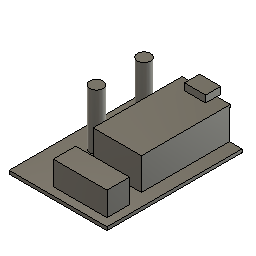
F000120 - Protoype Ingun Switch Case Assembly v8 (Autodesk Fusion 360 archive; units mm, degrees)
design "F000117 - Prototype Ingun Switch Breakout"
Autodesk Fusion 360 part; units mm, degrees
sketch "Sketch1" plane through (0, 0, 0) normal (0, 1, 0) x (1, 0, 0)
  line L0 (0, 0) -> (37, 0)
  line L1 (37, 0) -> (37, 51)
  line L2 (37, 51) -> (0, 51)
  line L3 (0, 51) -> (0, 0)
  line L4 (13.7, 3) -> (34, 3)
  line L5 (34, 3) -> (34, 11.5)
  line L6 (34, 11.5) -> (13.7, 11.5)
  line L7 (13.7, 11.5) -> (13.7, 3)
  line L8 (14, 17.75) -> (32.25, 17.75)
  line L9 (32.25, 17.75) -> (32.25, 51.35)
  line L10 (32.25, 51.35) -> (14, 51.35)
  line L11 (14, 51.35) -> (14, 17.75)
  line L12 (19.125, 47.15) -> (27.125, 47.15)
  line L13 (27.125, 47.15) -> (27.125, 52.85)
  line L14 (27.125, 52.85) -> (19.125, 52.85)
  line L15 (19.125, 52.85) -> (19.125, 47.15)
  circle A0 centre (9.5, 41.5) radius 2.5
  circle A1 centre (9.5, 23.5) radius 2.5
  dimension "d1" = 37
  dimension "d2" = 51
  dimension "d3" = 3
  dimension "d4" = 3
  dimension "d5" = 20.3
  dimension "d6" = 8.5
  dimension "d7" = 6.25
  dimension "d8" = 18.25
  dimension "d9" = 4.75
  dimension "d10" = 33.6
  dimension "d11" = 5.7
  dimension "d12" = 8
  dimension "d13" = 5.125
  dimension "d15" = 1.5
  dimension "d16" = 9.5
  dimension "d17" = 9.5
  dimension "d18" = 5
  dimension "d19" = 27.5
  constraint horizontal L0
  constraint vertical L1
  constraint horizontal L2
  constraint vertical L3
  constraint coincident L0.start L3.end
  constraint horizontal L4
  constraint vertical L5
  constraint horizontal L6
  constraint vertical L7
  constraint horizontal L8
  constraint vertical L9
  constraint horizontal L10
  constraint vertical L11
  constraint horizontal L12
  constraint vertical L13
  constraint horizontal L14
  constraint vertical L15
  constraint equal A0 A1
  constraint vertical A0.centre A1.centre
  measures "d1" distance of L0.start L0.end
  measures "d2" distance of L0.start L2.end
  measures "d3" distance of L0 L4
  measures "d4" distance of L1 L5
  measures "d5" distance of L4.start L4.end
  measures "d6" distance of L4.start L6.end
  measures "d7" distance of L6 L8
  measures "d8" distance of L8.start L8.end
  measures "d9" distance of L1 L9
  measures "d10" distance of L8.end L9.end
  measures "d11" distance of L12.start L14.end
  measures "d12" distance of L13.end L14.end
  measures "d13" distance of L11 L15
  measures "d15" distance of L10 L14
  measures "d16" distance of L2 A0.centre
  measures "d17" distance of L3 A0.centre
  measures "d18" diameter of A0
  measures "d19" distance of L2 A1.centre
extrude "Extrude1" add sketch "Sketch1" against normal blind 1.25 contours L0 L1 L2 L3 L8 L9 L11 | L2 L8 L9 L11 L12 L13 L15 | L2 L12 L13 L15 | L4 L5 L6 L7 | A0 | A1
extrude "Extrude2" add sketch "Sketch1" along normal blind 9 contours L4 L5 L6 L7
extrude "Extrude3" add sketch "Sketch1" along normal blind 11 contours L2 L8 L9 L11 L12 L13 L15 | L2 L12 L13 L15
sketch "Sketch3" plane through (0, 11, 0) normal (0, 1, 0) x (-1, 0, 0)
  line L0 (-32.25, -51) -> (-14, -51)
  line L1 (-14, -51) -> (-14, -17.75)
  line L2 (-14, -17.75) -> (-32.25, -17.75)
  line L3 (-32.25, -17.75) -> (-32.25, -51)
  line L4 (-14, -17.75) -> (-32.25, -17.75)
  line L5 (-32.25, -17.75) -> (-32.25, -51.35)
  line L6 (-32.25, -51.35) -> (-14, -51.35)
  line L7 (-14, -51.35) -> (-14, -17.75)
  dimension "d26" = 33.6
  dimension "d27" = 18.25
  constraint horizontal L4
  constraint vertical L5
  constraint horizontal L6
  constraint vertical L7
  constraint coincident L1.end L2.start
  measures "d26" distance of L2.end L5.end
  measures "d27" distance of L5.end L6.end
extrude "Extrude4" add sketch "Sketch3" along normal blind 1
sketch "Sketch4" plane through (0, 12, 0) normal (0, 1, 0) x (-1, 0, 0)
  line L0 (-14, -51.35) -> (-14, -17.75)
  line L1 (-14, -17.75) -> (-32.25, -17.75)
  line L2 (-32.25, -17.75) -> (-32.25, -51.35)
  line L3 (-32.25, -51.35) -> (-14, -51.35)
  line L4 (-19.125, -47.15) -> (-27.125, -47.15)
  line L5 (-27.125, -47.15) -> (-27.125, -52.85)
  line L6 (-27.125, -52.85) -> (-19.125, -52.85)
  line L7 (-19.125, -52.85) -> (-19.125, -47.15)
  line L8 (-32.25, -51.35) -> (-14, -51.35)
  dimension "d30" = 5.125
  dimension "d31" = 8
  dimension "d32" = 5.7
  dimension "d33" = 1.5
  constraint horizontal L4
  constraint vertical L5
  constraint horizontal L6
  constraint vertical L7
  measures "d30" distance of L0.start L7
  measures "d31" distance of L5.end L6.end
  measures "d32" distance of L4.start L6.end
  measures "d33" distance of L6 L8
extrude "Extrude5" add sketch "Sketch4" along normal blind 2.6 contours L3 L5 L6 L7 L8 | L3 L4 L5 L7 L8
extrude "Extrude6" add sketch "Sketch1" along normal blind 21 contours A0 | A1
sketch "Sketch6" plane through (0, -1.25, 0) normal (0, -1, 0) x (1, 0, 0)
  line L0 (0, 0) -> (0, -51)
  line L1 (0, -51) -> (37, -51)
  line L2 (37, -51) -> (37, 0)
  line L3 (37, 0) -> (0, 0)
  line L4 (4, -4) -> (33, -4)
  line L5 (33, -4) -> (33, -49)
  line L6 (33, -49) -> (4, -49)
  line L7 (4, -49) -> (4, -4)
  dimension "d38" = 2
  dimension "d39" = 4
  dimension "d41" = 4
  dimension "d42" = 4
  dimension "d45" = 29
  dimension "d46" = 45
  constraint horizontal L4
  constraint vertical L5
  constraint horizontal L6
  constraint vertical L7
  measures "d38" distance of L1 L6
  measures "d39" distance of L0 L7
  measures "d41" distance of L2 L5
  measures "d42" distance of L3 L4
  measures "d45" distance of L4.start L4.end
  measures "d46" distance of L4.start L6.end
extrude "Extrude7" [suppressed]

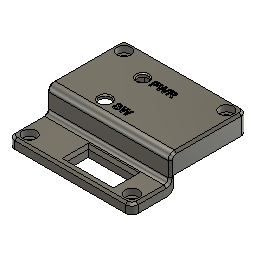
design "F000119 - Case Top"
Autodesk Fusion 360 part; units mm, degrees
sketch "Sketch1" plane through (0, 0, 0) normal (0, 1, 0) x (1, 0, 0)
  line L0 (0, 0) -> (59, 0)
  line L1 (59, 0) -> (59, 56.2)
  line L2 (59, 56.2) -> (0, 56.2)
  line L3 (0, 56.2) -> (0, 0)
  line L4 (23.85, 14.25) -> (45.85, 14.25)
  line L5 (45.85, 14.25) -> (45.85, 4.25)
  line L6 (45.85, 4.25) -> (23.85, 4.25)
  line L7 (23.85, 4.25) -> (23.85, 14.25)
  line L8 (0, 18.25) -> (59, 18.25)
  line L9 (0, 19.85) -> (59, 19.85)
  dimension "d1" = 59
  dimension "d2" = 56.2
  dimension "d3" = 13.15
  dimension "d4" = 10
  dimension "d5" = 22
  dimension "d6" = 4.25
  dimension "d11" = 4
  dimension "d12" = 1.6
  constraint horizontal L0
  constraint vertical L1
  constraint horizontal L2
  constraint vertical L3
  constraint coincident L0.start L3.end
  constraint horizontal L4
  constraint vertical L5
  constraint horizontal L6
  constraint vertical L7
  constraint coincident L3 L8.start
  constraint coincident L1 L8.end
  constraint perpendicular L1 L8
  constraint coincident L3 L9.start
  constraint coincident L1 L9.end
  constraint perpendicular L1 L9
  measures "d1" distance of L0.start L0.end
  measures "d2" distance of L0.start L2.end
  measures "d3" distance of L1 L5
  measures "d4" distance of L4.end L5.end
  measures "d5" distance of L4.start L4.end
  measures "d11" distance of L4 L8
  measures "d12" distance of L8 L9
  measures "d24" distance of L0.start
  measures "d34" distance of L0.start
  measures "d51" distance of L0.start
extrude "Extrude1" add sketch "Sketch1" against normal blind 4.6 contours L0 L1 L3 L8 | L1 L3 L8 L9
extrude "Extrude2" add sketch "Sketch1" along normal blind 10.45 contours L1 L3 L8 L9
sketch "Sketch2" plane through (0, 10.45, 0) normal (0, 1, 0) x (-1, 0, 0)
  line L0 (0, -18.25) -> (-59, -18.25)
  line L1 (-59, -18.25) -> (-59, -19.85)
  line L2 (-59, -19.85) -> (0, -19.85)
  line L3 (0, -19.85) -> (0, -18.25)
  line L4 (0, -18.25) -> (-59, -18.25)
  line L5 (-59, -18.25) -> (-59, -55.2)
  line L6 (-59, -55.2) -> (0, -55.2)
  line L7 (0, -55.2) -> (0, -18.25)
  dimension "d15" = 36.95
  dimension "d16" = 59
  constraint horizontal L4
  constraint vertical L5
  constraint horizontal L6
  constraint vertical L7
  constraint coincident L0.start L3.end
  measures "d15" distance of L0.start L6.end
  measures "d16" distance of L5.end L6.end
extrude "Extrude3" add sketch "Sketch2" along normal blind 1.6
fillet "Fillet1" radius 2 1 edges at (29.5, 0, -18.25)
fillet "Fillet2" radius 3 1 edges at (29.5, -4.6, -19.85)
fillet "Fillet3" radius 3 1 edges at (29.5, 12.05, -18.25)
sketch "Sketch3" plane through (0, 10.45, 0) normal (0, -1, 0) x (1, 0, 0)
  line L0 (59, -19.85) -> (0, -19.85)
  line L1 (0, -19.85) -> (0, -55.2)
  line L2 (0, -55.2) -> (59, -55.2)
  line L3 (59, -55.2) -> (59, -19.85)
  line L4 (57.4, -53.6) -> (1.6, -53.6)
  line L5 (1.6, -53.6) -> (1.6, -19.85)
  line L6 (1.6, -19.85) -> (57.4, -19.85)
  line L7 (57.4, -19.85) -> (57.4, -53.6)
  line L8 (1.6, -53.6) -> (1.6, -55.2)
  line L9 (57.4, -53.6) -> (57.4, -55.2)
  line L10 (3.2, -53.6) -> (3.2, -19.85)
  line L11 (55.8, -19.85) -> (55.8, -53.6)
  line L12 (3.2, -52) -> (55.8, -52)
  line L13 (44.25, -52) -> (44.25, -53.6)
  line L14 (24, -52) -> (24, -53.6)
  dimension "d23" = 1.6
  dimension "d24" = 1.6
  dimension "d25" = 1.6
  dimension "d73" = 1.6
  dimension "d74" = 1.6
  dimension "d77" = 1.6
  dimension "d83" = 22.4
  dimension "d84" = 13.15
  constraint horizontal L4
  constraint vertical L5
  constraint horizontal L6
  constraint vertical L7
  constraint horizontal L0.start L6.end
  constraint coincident L2 L8.end
  constraint perpendicular L2 L8
  constraint coincident L2 L9.end
  constraint perpendicular L2 L9
  constraint parallel L5 L10
  constraint parallel L7 L11
  constraint coincident L0 L10.end
  constraint coincident L4 L10.start
  constraint coincident L6 L11.start
  constraint coincident L4 L11.end
  constraint coincident L10 L12.start
  constraint coincident L11 L12.end
  constraint perpendicular L11 L12
  constraint coincident L12 L13.start
  constraint coincident L4 L13.end
  constraint perpendicular L4 L13
  constraint coincident L12 L14.start
  constraint coincident L4 L14.end
  constraint perpendicular L4 L14
  measures "d23" distance of L3 L7
  measures "d24" distance of L1 L5
  measures "d25" distance of L2 L4
  measures "d73" distance of L5 L10
  measures "d74" distance of L7 L11
  measures "d77" distance of L4 L12
  measures "d83" distance of L4.end L14
  measures "d84" distance of L4.start L13
extrude "Extrude4" add sketch "Sketch3" along normal blind 7.7 contours L0 L2 L3 L7 L9 | L0 L1 L2 L5 L8
extrude "Extrude10" add sketch "Sketch3" along normal blind 8.7 contours L0 L4 L6 L7 L11 | L0 L4 L5 L6 L10 | L4 L11 L12 L13 | L4 L10 L12 L14
sketch "Sketch4" plane through (0, 0, -55.2) normal (0, 0, -1) x (-1, 0, 0)
  line L0 (-57.4, 10.45) -> (-1.6, 10.45)
  line L1 (-1.6, 10.45) -> (-1.6, 2.75)
  line L2 (-1.6, 2.75) -> (0, 2.75)
  line L3 (0, 2.75) -> (0, 12.05)
  line L4 (0, 12.05) -> (-59, 12.05)
  line L5 (-59, 12.05) -> (-59, 2.75)
  line L6 (-59, 2.75) -> (-57.4, 2.75)
  line L7 (-57.4, 2.75) -> (-57.4, 10.45)
  line L8 (-59, 12.05) -> (0, 12.05)
  line L9 (0, 12.05) -> (0, 2.75)
  line L10 (0, 2.75) -> (-59, 2.75)
  line L11 (-59, 2.75) -> (-59, 12.05)
  line L12 (-38.25, 12.05) -> (-30, 12.05)
  line L13 (-30, 12.05) -> (-30, 2.75)
  line L14 (-30, 2.75) -> (-38.25, 2.75)
  line L15 (-38.25, 2.75) -> (-38.25, 12.05)
  line L16 (-38.25, 5.95) -> (-30, 5.95)
  dimension "d28" = 20.75
  dimension "d29" = 30
  dimension "d40" = 3.2
  constraint horizontal L8
  constraint vertical L9
  constraint horizontal L10
  constraint vertical L11
  constraint coincident L2.end L3.start
  constraint coincident L4.end L5.start
  constraint horizontal L12
  constraint vertical L13
  constraint horizontal L14
  constraint vertical L15
  constraint coincident L10 L13.end
  constraint coincident L8 L12.start
  constraint coincident L15 L16.start
  constraint coincident L13 L16.end
  constraint perpendicular L13 L16
  measures "d28" distance of L11 L15
  measures "d29" distance of L9 L13
  measures "d40" distance of L14 L16
extrude "Extrude5" add sketch "Sketch4" against normal blind 1.6 contours L0 L7 L10 L15 | L0 L1 L10 L13
sketch "Sketch5" plane through (0, 12.05, 0) normal (0, 1, 0) x (-1, 0, 0)
  line L0 (0, -21.25) -> (-59, -21.25)
  line L1 (-59, -21.25) -> (-59, -55.2)
  line L2 (-59, -55.2) -> (0, -55.2)
  line L3 (0, -55.2) -> (0, -21.25)
  circle A0 centre (-20.5, -25.6) radius 2.75
  circle A1 centre (-20.5, -43.6) radius 2.6
  dimension "d32" = 5.5
  dimension "d33" = 5.2
  dimension "d34" = 20.5
  dimension "d36" = 29.6
  dimension "d39" = 18
  constraint vertical A0.centre A1.centre
  measures "d32" diameter of A0
  measures "d33" diameter of A1
  measures "d34" distance of L3 A1.centre
  measures "d36" distance of L2 A0.centre
  measures "d39" distance of A0.centre A1.centre
extrude "Extrude6" cut sketch "Sketch5" against normal blind 19 contours A0 | A1
extrude "Extrude7" add sketch "Sketch4" against normal blind 1.6 contours L0 L13 L15 L16
sketch "Sketch6" plane through (0, 10.45, 0) normal (0, -1, 0) x (1, 0, 0)
  line L0 (24, -53.6) -> (44.25, -53.6)
  line L1 (55.8, -19.85) -> (3.2, -19.85)
  circle A0 centre (20.5, -43.6) radius 2.6
  circle A1 centre (20.5, -25.6) radius 2.75
  line L2 (1.6, -45.2) -> (10, -45.2)
  line L3 (10, -45.2) -> (10, -53.6)
  line L4 (57.4, -45.2) -> (49, -45.2)
  line L5 (49, -45.2) -> (49, -53.6)
  line L6 (44.25, -53.6) -> (44.25, -52)
  line L7 (44.25, -52) -> (55.8, -52)
  line L8 (55.8, -52) -> (55.8, -19.85)
  line L9 (3.2, -19.85) -> (3.2, -52)
  line L10 (3.2, -52) -> (24, -52)
  line L11 (24, -52) -> (24, -53.6)
  dimension "d43" = 8.4
  dimension "d44" = 8.4
  dimension "d45" = 8.4
  dimension "d46" = 8.4
  constraint coincident L0 L3.end
  constraint perpendicular L0 L3
  constraint coincident L0 L5.end
  constraint perpendicular L0 L5
  measures "d43" distance of L2.end L3.end
  measures "d44" distance of L2.start L2.end
  measures "d45" distance of L4.start L4.end
  measures "d46" distance of L4.end L5.end
extrude "Extrude8" add sketch "Sketch6" along normal blind 8.7 contours L2 L3 L9 L10 | L4 L5 L7 L8
fillet "Fillet4" radius 3 8 edges at (10, 6.1, -52) (10, 6.1, -45.2) (3.2, 6.1, -45.2) (49, 6.1, -52) (49, 6.1, -45.2) (55.8, 6.1, -45.2) (55.8, 6.1, -19.85) (3.2, 6.1, -19.85)
sketch "Sketch7" plane through (0, 12.05, 0) normal (0, 1, 0) x (-1, 0, 0)
  circle A0 centre (-20.5, -25.6) radius 2.75
  circle A1 centre (-20.5, -43.6) radius 2.6
  line L0 (0, -21.25) -> (-59, -21.25)
  line L1 (-59, -21.25) -> (-59, -55.2)
  line L2 (-59, -55.2) -> (0, -55.2)
  line L3 (0, -55.2) -> (0, -21.25)
  point P0 (-5, -50.2)
  point P1 (-54, -50.2)
  dimension "d50" = 5
  dimension "d51" = 5
  dimension "d52" = 5
  constraint horizontal P0 P1
  measures "d50" distance of L2 P0
  measures "d51" distance of L3 P0
  measures "d52" distance of L1 P1
sketch "Sketch8" plane through (0, 0, 0) normal (0, 1, 0) x (-1, 0, 0)
  line L0 (-59, -16.25) -> (0, -16.25)
  line L1 (0, -16.25) -> (0, 0)
  line L2 (0, 0) -> (-59, 0)
  line L3 (-59, 0) -> (-59, -16.25)
  line L4 (-45.85, -4.25) -> (-23.85, -4.25)
  line L5 (-23.85, -4.25) -> (-23.85, -14.25)
  line L6 (-23.85, -14.25) -> (-45.85, -14.25)
  line L7 (-45.85, -14.25) -> (-45.85, -4.25)
  point P0 (-5, -5)
  point P1 (-54, -5)
  dimension "d58" = 5
  dimension "d59" = 5
  dimension "d60" = 5
  constraint horizontal P0 P1
  measures "d58" distance of L1 P0
  measures "d59" distance of L2 P0
  measures "d60" distance of L3 P1
hole "Hole1" at (5, 12.05, -50.2) at (54, 12.05, -50.2) direction (0, -1, 0) diameter 3.4 depth 14 tip angle 180 counterbore diameter 6.5 counterbore depth 3
hole "Hole2" at (5, 0, -5) at (54, 0, -5) direction (0, -1, 0) diameter 3.4 depth 10 tip angle 180 counterbore diameter 6.5 counterbore depth 3
fillet "Fillet5" radius 3 4 edges at (59, 7.4, -55.2) (0, 7.4, -55.2) (0, -2.3, 0) (59, -2.3, 0)
chamfer "Chamfer1" distance 1 angle 45 16 edges at (0, 11.1713, -19.1287) (0, 5.525, -18.25) (0, 0.5858, -17.6642) (0, 0, -9.625) (0.8787, 0, -0.8787) (29.5, 0, 0) (58.1213, 0, -0.8787) (59, 0, -9.625) (59, 0.5858, -17.6642) (59, 5.525, -18.25) (59, 11.1713, -19.1287) (59, 12.05, -36.725) (58.1213, 12.05, -54.3213) (29.5, 12.05, -55.2) (0.8787, 12.05, -54.3213) (0, 12.05, -36.725)
chamfer "Chamfer2" distance 1.25 angle 45 4 edges at (34.85, 0, -4.25) (23.85, 0, -9.25) (34.85, 0, -14.25) (45.85, 0, -9.25)
fillet "Fillet6" radius 0.5 2 edges at (22.9241, 12.05, -42.6598) (23.0639, 12.05, -24.6056)
sketch "Sketch9" plane through (0, 12.05, 0) normal (0, 1, 0) x (-1, 0, 0)
  circle A0 centre (-20.5, -43.6) radius 3.1
  circle A1 centre (-5, -50.2) radius 3.25
  circle A2 centre (-54, -50.2) radius 3.25
  line L0 (-58, -21.25) -> (-58, -52.2)
  arc A3 (-58, -52.2) -> (-56, -54.2) centre (-56, -52.2) ccw
  line L1 (-56, -54.2) -> (-3, -54.2)
  arc A4 (-3, -54.2) -> (-1, -52.2) centre (-3, -52.2) ccw
  line L2 (-1, -52.2) -> (-1, -21.25)
  line L3 (-1, -21.25) -> (-58, -21.25)
  circle A5 centre (-20.5, -25.6) radius 3.25
  line L4 (-25, -42) -> (-36.1861, -41.9973) construction
  line L5 (-36.1861, -41.9973) -> (-36.1872, -46.8542) construction
  line L6 (-36.1872, -46.8542) -> (-25.0012, -46.8569) construction
  line L7 (-25.0012, -46.8569) -> (-25, -42) construction
  line L8 (-25, -23.9666) -> (-32.7185, -23.9597) construction
  line L9 (-32.7185, -23.9597) -> (-32.7229, -28.7859) construction
  line L10 (-32.7229, -28.7859) -> (-25.0043, -28.7928) construction
  line L11 (-25.0043, -28.7928) -> (-25, -23.9666) construction
  text T0 "PWR" font "Arial" height 4.8569 bold align ink ink in box 0 x 0 at (-25, -42) x (-1, 0.000243) y (-0.000243, -1) spacing 1 height is em
  text T1 "SW" font "Arial" height 4.8262 bold align ink ink in box 0 x 0 at (-25, -23.9666) x (-1, 0.000895) y (-0.000895, -1) spacing 1 height is em
  constraint perpendicular L4 L5
  constraint parallel L4 L6
  constraint parallel L5 L7
  constraint perpendicular L8 L9
  constraint parallel L8 L10
  constraint parallel L9 L11
  constraint vertical L4.start L8.start
extrude "Extrude9" cut sketch "Sketch9" against normal blind 0.4 text T0 T1
equation "d3 = 13.5 mm - 0.35 mm"
equation "d6 = 5.1 mm - 0.5 mm - 0.35 mm"
equation "d13 = 4.35 mm + 1.6 mm + 4.5 mm"
equation "d15 = 36.35 mm + 0.75 mm - 0.15 mm"
equation "d26 = 3.2 mm + 4.5 mm"
equation "d28 = 20.875 mm - 0.125 mm"
equation "d34 = 22.958 mm - 1.458 mm - 1 mm"
equation "d36 = 27.691 mm + 1.909 mm"
equation "d44 = 5 mm - 1.6 mm + 5 mm"

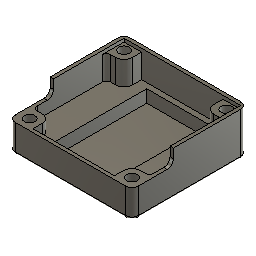
design "F000118 - Case Bottom"
Autodesk Fusion 360 part; units mm, degrees
sketch "Sketch1" plane through (0, 0, 0) normal (0, 1, 0) x (1, 0, 0)
  line L0 (0, 0) -> (59, 0)
  line L1 (59, 0) -> (59, 55.2)
  line L2 (59, 55.2) -> (0, 55.2)
  line L3 (0, 55.2) -> (0, 0)
  line L4 (15, 51.1) -> (45, 51.1)
  line L5 (45, 51.1) -> (45, 5.1)
  line L6 (45, 5.1) -> (15, 5.1)
  line L7 (15, 5.1) -> (15, 51.1)
  line L8 (10, 53.6) -> (49, 53.6)
  line L9 (49, 1.6) -> (10, 1.6)
  circle A0 centre (5, 5) radius 3
  circle A1 centre (54, 5) radius 3
  circle A2 centre (5, 50.2) radius 3
  circle A3 centre (54, 50.2) radius 3
  line L10 (6, 45.2) -> (3.6, 45.2)
  line L11 (1.6, 43.2) -> (1.6, 12)
  line L12 (3.6, 10) -> (6, 10)
  line L13 (53, 45.2) -> (55.4, 45.2)
  line L14 (57.4, 43.2) -> (57.4, 12)
  line L15 (55.4, 10) -> (53, 10)
  arc A4 (3.6, 45.2) -> (1.6, 43.2) centre (3.6, 43.2) ccw
  arc A5 (57.4, 43.2) -> (55.4, 45.2) centre (55.4, 43.2) ccw
  arc A6 (55.4, 10) -> (57.4, 12) centre (55.4, 12) ccw
  arc A7 (1.6, 12) -> (3.6, 10) centre (3.6, 12) ccw
  line L16 (10, 53.6) -> (10, 49.2)
  line L17 (10, 6) -> (10, 1.6)
  arc A8 (6, 45.2) -> (10, 49.2) centre (6, 49.2) ccw
  arc A9 (10, 6) -> (6, 10) centre (6, 6) ccw
  line L18 (49, 53.6) -> (49, 49.2)
  line L19 (49, 6) -> (49, 1.6)
  arc A10 (49, 49.2) -> (53, 45.2) centre (53, 49.2) ccw
  arc A11 (53, 10) -> (49, 6) centre (53, 6) ccw
  dimension "d3" = 30
  dimension "d4" = 46
  dimension "d5" = 39
  dimension "d6" = 52
  dimension "d7" = 2.5
  dimension "d8" = 4
  dimension "d11" = 1.6
  dimension "d12" = 1.6
  dimension "d17" = 6
  dimension "d18" = 5
  dimension "d19" = 5
  dimension "d20" = 5
  dimension "d21" = 5
  dimension "d34" = 59
  dimension "d35" = 59
  dimension "d50" = 5
  dimension "d51" = 5
  dimension "d52" = 1.6
  dimension "d53" = 1.6
  dimension "d54" = 2
  dimension "d56" = 5
  dimension "d57" = 4
  dimension "d58" = 4
  dimension "d59" = 5
  dimension "d60" = 5
  dimension "d61" = 5
  dimension "d62" = 5
  dimension "d63" = 5
  dimension "d64" = 4
  dimension "d66" = 15
  constraint horizontal L0
  constraint vertical L1
  constraint horizontal L2
  constraint vertical L3
  constraint coincident L0.start L3.end
  constraint horizontal L4
  constraint vertical L5
  constraint horizontal L6
  constraint vertical L7
  constraint horizontal L8
  constraint horizontal L9
  constraint equal A0 A1
  constraint horizontal A0.centre A1.centre
  constraint equal A1 A3
  constraint equal A1 A2
  constraint horizontal A2.centre A3.centre
  constraint vertical A1.centre A3.centre
  constraint vertical A0.centre A2.centre
  constraint perpendicular L10 L11
  constraint perpendicular L11 L12
  constraint perpendicular L13 L14
  constraint tangent L10 A4
  constraint tangent L11 A4
  constraint tangent L13 A5
  constraint tangent L14 A5
  constraint equal A4 A5
  constraint tangent L14 A6
  constraint tangent L15 A6
  constraint equal A4 A6
  constraint tangent L11 A7
  constraint tangent L12 A7
  constraint equal A4 A7
  constraint perpendicular L8 L16
  constraint perpendicular L9 L17
  constraint tangent L10 A8
  constraint tangent L16 A8
  constraint tangent L12 A9
  constraint tangent L17 A9
  constraint perpendicular L13 L18
  constraint perpendicular L9 L19
  constraint horizontal L15
  constraint tangent L13 A10
  constraint tangent L18 A10
  constraint tangent L15 A11
  constraint tangent L19 A11
  constraint equal A10 A11
  measures "d3" distance of L5.end L6.end
  measures "d4" distance of L4.start L6.end
  measures "d5" distance of L8.start L8.end
  measures "d6" distance of L8.start L9.end
  measures "d7" distance of L4 L8
  measures "d11" distance of L0 L9
  measures "d12" distance of L2 L8
  measures "d17" diameter of A0
  measures "d18" distance of L3 A0.centre
  measures "d19" distance of L1 A1.centre
  measures "d20" distance of L0 A1.centre
  measures "d21" distance of L2 A2.centre
  measures "d34" distance of L0.start L0.end
  measures "d50" distance of A2.centre L10
  measures "d51" distance of A1.centre L15
  measures "d52" distance of L1 L14
  measures "d53" distance of L3 L11
  measures "d54" radius of A4
  measures "d56" distance of A0.centre L17
  measures "d57" radius of A8
  measures "d58" radius of A9
  measures "d59" distance of A0.centre L12
  measures "d60" distance of A1.centre L19
  measures "d61" distance of A3.centre L18
  measures "d62" distance of A3.centre L13
  measures "d63" distance of A2.centre L16
  measures "d64" radius of A10
  measures "d66" distance of L3 L7
extrude "Extrude1" add sketch "Sketch1" against normal blind 1.6 contours L0 L1 L2 L3 | L4 L5 L6 L7 | L8 L9 L10 L11 L12 L13 L14 L15 A4 A5 A6 A7 L16 L17 A8 A9 L18 L19 A10 A11 | A0 | A1 | A2 | A3
extrude "Extrude2" add sketch "Sketch1" along normal blind 6 contours L8 L9 L10 L11 L12 L13 L14 L15 A4 A5 A6 A7 L16 L17 A8 A9 L18 L19 A10 A11
extrude "Extrude3" add sketch "Sketch1" along normal blind 11.65 contours L0 L1 L2 L3 | A0 | A1 | A2 | A3
sketch "Sketch2" plane through (0, 11.65, 0) normal (0, 1, 0) x (-1, 0, 0)
  line L0 (-49, -1.6) -> (-10, -1.6)
  line L1 (-10, -53.6) -> (-49, -53.6)
  line L2 (0, -55.2) -> (0, 0)
  line L3 (0, 0) -> (-59, 0)
  line L4 (-59, 0) -> (-59, -55.2)
  line L5 (-59, -55.2) -> (0, -55.2)
  line L6 (-59, -55.2) -> (0, -55.2)
  line L7 (0, -55.2) -> (0, 0)
  line L8 (-59, 0) -> (-59, -55.2)
  line L9 (0, 0) -> (-59, 0)
  line L10 (0, -19.85) -> (-10.5, -19.85)
  line L11 (0, -19.85) -> (0, -55.2)
  line L12 (0, -55.2) -> (-59, -55.2)
  line L13 (-59, -55.2) -> (-59, -19.85)
  line L14 (-59, -19.85) -> (-49.5, -19.85)
  arc A0 (-55.4, -10) -> (-57.4, -12) centre (-55.4, -12) ccw
  line L15 (-55.4, -10) -> (-53, -10)
  arc A1 (-53, -10) -> (-49, -6) centre (-53, -6) ccw
  line L16 (-49, -6) -> (-49, -1.6)
  line L17 (-10, -1.6) -> (-10, -6)
  arc A2 (-10, -6) -> (-6, -10) centre (-6, -6) ccw
  line L18 (-6, -10) -> (-3.6, -10)
  arc A3 (-1.6, -12) -> (-3.6, -10) centre (-3.6, -12) ccw
  line L19 (-1.6, -12) -> (-1.6, -43.2)
  arc A4 (-3.6, -45.2) -> (-1.6, -43.2) centre (-3.6, -43.2) ccw
  line L20 (-3.6, -45.2) -> (-6, -45.2)
  arc A5 (-6, -45.2) -> (-10, -49.2) centre (-6, -49.2) ccw
  line L21 (-10, -49.2) -> (-10, -53.6)
  line L22 (-49, -53.6) -> (-49, -49.2)
  arc A6 (-49, -49.2) -> (-53, -45.2) centre (-53, -49.2) ccw
  line L23 (-53, -45.2) -> (-55.4, -45.2)
  arc A7 (-57.4, -43.2) -> (-55.4, -45.2) centre (-55.4, -43.2) ccw
  line L24 (-57.4, -43.2) -> (-57.4, -12)
  point P0 (-5, -50.2)
  point P1 (-54, -50.2)
  point P2 (-54, -5)
  point P3 (-5, -5)
  dimension "d36" = 5
  dimension "d37" = 5
  dimension "d38" = 5
  dimension "d39" = 5
  dimension "d40" = 19.85
  dimension "d41" = 19.85
  constraint horizontal P0 P1
  constraint vertical P1 P2
  constraint horizontal P2 P3
  constraint vertical P0 P3
  constraint coincident L7 L10.start
  constraint coincident L2.start L5.end
  constraint coincident L4.end L5.start
  constraint coincident L4 L13.end
  constraint perpendicular L5 L13
  measures "d36" distance of P0 L6
  measures "d37" distance of P0 L7
  measures "d38" distance of P2 L8
  measures "d39" distance of P2 L9
  measures "d40" distance of L9 L10
  measures "d41" distance of L9 L14
hole "Hole2" at (5, 11.65, -50.2) at (54, 11.65, -50.2) at (54, 11.65, -5) at (5, 11.65, -5) direction (0, -1, 0) diameter 5.055 depth 10 tip angle 180
sketch "Sketch3" plane through (0, 11.65, 0) normal (0, 1, 0) x (-1, 0, 0)
  circle A0 centre (-54, -5) radius 2.5275
  circle A1 centre (-5, -50.2) radius 2.5275
  circle A2 centre (-54, -50.2) radius 2.5275
  circle A3 centre (-5, -5) radius 2.5275
  line L0 (-49, -1.6) -> (-10, -1.6)
  line L1 (-10, -53.6) -> (-49, -53.6)
  line L2 (0, -55.2) -> (0, 0)
  line L3 (0, 0) -> (-59, 0)
  line L4 (-59, 0) -> (-59, -55.2)
  line L5 (-59, -55.2) -> (0, -55.2)
  arc A4 (-55.4, -10) -> (-57.4, -12) centre (-55.4, -12) ccw
  line L6 (-55.4, -10) -> (-53, -10)
  arc A5 (-53, -10) -> (-49, -6) centre (-53, -6) ccw
  line L7 (-49, -6) -> (-49, -1.6)
  line L8 (-10, -1.6) -> (-10, -6)
  arc A6 (-10, -6) -> (-6, -10) centre (-6, -6) ccw
  line L9 (-6, -10) -> (-3.6, -10)
  arc A7 (-1.6, -12) -> (-3.6, -10) centre (-3.6, -12) ccw
  line L10 (-1.6, -12) -> (-1.6, -43.2)
  arc A8 (-3.6, -45.2) -> (-1.6, -43.2) centre (-3.6, -43.2) ccw
  line L11 (-3.6, -45.2) -> (-6, -45.2)
  arc A9 (-6, -45.2) -> (-10, -49.2) centre (-6, -49.2) ccw
  line L12 (-10, -49.2) -> (-10, -53.6)
  line L13 (-49, -53.6) -> (-49, -49.2)
  arc A10 (-49, -49.2) -> (-53, -45.2) centre (-53, -49.2) ccw
  line L14 (-53, -45.2) -> (-55.4, -45.2)
  arc A11 (-57.4, -43.2) -> (-55.4, -45.2) centre (-55.4, -43.2) ccw
  line L15 (-57.4, -43.2) -> (-57.4, -12)
extrude "Extrude4" add sketch "Sketch2" along normal blind 7.35 contours L1 L2 L4 L5 L6 L7 L8 L10 L11 L12 L13 L14 L19 A4 L20 A5 L21 L22 A6 L23 A7 L24
sketch "Sketch4" plane through (0, 19, 0) normal (0, 1, 0) x (-1, 0, 0)
  line L0 (0, -19.85) -> (-1.6, -19.85)
  line L1 (-10, -53.6) -> (-49, -53.6)
  line L2 (-57.4, -19.85) -> (-59, -19.85)
  line L3 (-59, -19.85) -> (-59, -55.2)
  line L4 (-59, -55.2) -> (0, -55.2)
  line L5 (0, -55.2) -> (0, -19.85)
  line L6 (0, -55.2) -> (-59, -55.2)
  line L7 (0, -19.85) -> (0, -55.2)
  line L8 (-59, -55.2) -> (-59, -19.85)
  line L9 (-1.6, -19.85) -> (-1.6, -43.2)
  arc A0 (-3.6, -45.2) -> (-1.6, -43.2) centre (-3.6, -43.2) ccw
  line L10 (-3.6, -45.2) -> (-6, -45.2)
  arc A1 (-6, -45.2) -> (-10, -49.2) centre (-6, -49.2) ccw
  line L11 (-10, -49.2) -> (-10, -53.6)
  line L12 (-49, -53.6) -> (-49, -49.2)
  arc A2 (-49, -49.2) -> (-53, -45.2) centre (-53, -49.2) ccw
  line L13 (-53, -45.2) -> (-55.4, -45.2)
  arc A3 (-57.4, -43.2) -> (-55.4, -45.2) centre (-55.4, -43.2) ccw
  line L14 (-57.4, -43.2) -> (-57.4, -19.85)
  line L15 (-57.4, -43.2) -> (-57.4, -53.6)
  line L16 (-57.4, -53.6) -> (-49, -53.6)
  line L17 (-1.6, -43.2) -> (-1.6, -53.6)
  line L18 (-1.6, -53.6) -> (-10, -53.6)
  point P0 (-5, -50.2)
  point P1 (-54, -50.2)
  point P2 (-5, -50.2)
  point P3 (-5, -50.2)
  dimension "d44" = 5
  dimension "d45" = 5
  dimension "d46" = 5
  dimension "d69" = 1.6
  dimension "d70" = 1.6
  constraint coincident P3 P2
  constraint horizontal P1 P3
  constraint coincident A3.start L14.start
  constraint tangent A3 L15
  constraint coincident L12 L1.end
  constraint perpendicular L12 L16
  constraint coincident L9.end A0.end
  constraint tangent A0 L17
  constraint coincident L11 L1.start
  constraint perpendicular L11 L18
  measures "d44" distance of P3 L6
  measures "d45" distance of P3 L7
  measures "d46" distance of P1 L8
  measures "d69" distance of L6 L16
  measures "d70" distance of L4 L18
extrude "Extrude5" cut sketch "Sketch4" against normal blind 1.6 contours A0 L10 A1 L11 L17 L18 | L12 A2 L13 A3 L15 L16
hole "Hole3" at (5, 19, -50.2) at (54, 19, -50.2) direction (0, -1, 0) diameter 5.055 depth 11.6 tip angle 180
fillet "Fillet1" radius 3 2 edges at (58.2, 11.65, -19.85) (0.8, 11.65, -19.85)
fillet "Fillet2" radius 3 4 edges at (0, 5.025, 0) (59, 5.025, 0) (59, 8.7, -55.2) (0, 8.7, -55.2)
fillet "Fillet3" radius 1 8 edges at (0.8787, -1.6, -54.3213) (29.5, -1.6, -55.2) (58.1213, -1.6, -54.3213) (59, -1.6, -27.6) (58.1213, -1.6, -0.8787) (29.5, -1.6, 0) (0.8787, -1.6, -0.8787) (0, -1.6, -27.6)
sketch "Sketch5" plane through (0, 0, 0) normal (-1, 0, 0) x (0, 0, 1)
  line L0 (-52.2, -0.6) -> (-3, -0.6)
  line L1 (-3, -0.6) -> (-3, 11.65)
  line L2 (-3, 11.65) -> (-16.85, 11.65)
  arc A0 (-19.85, 14.65) -> (-16.85, 11.65) centre (-16.85, 14.65) ccw
  line L3 (-19.85, 14.65) -> (-19.85, 19)
  line L4 (-19.85, 19) -> (-52.2, 19)
  line L5 (-52.2, 19) -> (-52.2, -0.6)
  line L6 (-50, 9.9) -> (-30.9106, 9.9) construction
  line L7 (-30.9106, 9.9) -> (-30.9106, 14.9) construction
  line L8 (-30.9106, 14.9) -> (-50, 14.9) construction
  line L9 (-50, 14.9) -> (-50, 9.9) construction
  line L10 (-50, 3.9) -> (-22.1777, 3.9) construction
  line L11 (-22.1777, 3.9) -> (-22.1777, 8.9) construction
  line L12 (-22.1777, 8.9) -> (-50, 8.9) construction
  line L13 (-50, 8.9) -> (-50, 3.9) construction
  dimension "d73" = 4.5
  dimension "d74" = 10.5
  text T0 "F000120" font "Arial" height 5 align ink ink in box 0 x 0 at (-50, 9.9) x (1, 0) y (0, 1) spacing 1 height is em
  text T1 "Ingun Switch" font "Arial" height 5 align ink ink in box 0 x 0 at (-50, 3.9) x (1, 0) y (0, 1) spacing 1 height is em
  constraint perpendicular L6 L7
  constraint parallel L6 L8
  constraint parallel L7 L9
  constraint perpendicular L10 L11
  constraint parallel L10 L12
  constraint parallel L11 L13
  measures "d73" vertical distance of L0.start L10.start
  measures "d74" vertical distance of L0.start L6.start
extrude "Extrude6" cut sketch "Sketch5" against normal blind 0.4 text T0 T1
equation "d26 = 13 mm - 1.75 mm + 3.4 mm - 3 mm"
equation "d42 = 6 mm + 1.75 mm - 3.4 mm + 3 mm"
